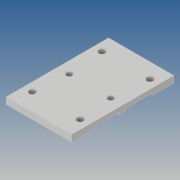
# Autodesk Inventor part: attache_exterieur
Saved by Autodesk Inventor 2019 (Build 230136000, 136)
## iProperties
Created: 2020-07-07
Part Number: attache_exterieur
Material: Générique
Document SubType Name: Modeling
Designer: Theo
Density: 1 g/cm^3
Appearance: Par défaut
Author: Theo
Autodesk Inventor part; units mm, degrees
ref_plane "YZ Plane" through (0, 0, 0) normal (1, 0, 0) x (0, 1, 0)
ref_plane "XZ Plane" through (0, 0, 0) normal (0, 1, 0) x (-1, 0, 0)
ref_plane "XY Plane" through (0, 0, 0) normal (0, 0, 1) x (1, 0, 0)
sketch "Esquisse1" plane through (0, 0, 0) normal (0, 1, 0) x (-1, 0, 0)
  line L0 (0, 0) -> (-60, 0)
  line L1 (-60, 0) -> (-60, 94)
  line L2 (-60, 94) -> (0, 94)
  line L3 (0, 94) -> (0, 0)
  dimension "d0" = 60
  dimension "d1" = 94
  constraints: 8 end point, 2 parallel, 1 horizontal, 1 perpendicular
  measures "d0" distance of L0.start L0.end
  measures "d1" distance of L2.end L0.start
extrude "Extrusion1" add sketch "Esquisse1" along normal blind 6
sketch "Esquisse2" plane through (0, 6, 0) normal (0, 1, 0) x (1, 0, 0)
  line L0 (0, -94) -> (60, -94) projected
  line L1 (60, 0) -> (0, 0) projected
  line L2 (0, 0) -> (0, -94) projected
  line L3 (60, -94) -> (60, 0) projected
  point P0 (8, -78)
  point P1 (52, -78)
  point P2 (52, -14)
  point P3 (8, -14)
  dimension "d4" = 16
  dimension "d5" = 14
  dimension "d6" = 8
  dimension "d7" = 8
  constraints: 2 horizontal alignment, 2 vertical alignment
  measures "d4" distance from line of L0 point (8, -78)
  measures "d5" distance from line of L1 point (8, -14)
  measures "d6" distance from line of L2 point (8, -78)
  measures "d7" distance from line of L3 point (52, -78)
hole "Perçage1" at (8, 6, 78) at (52, 6, 78) at (52, 6, 14) at (8, 6, 14) direction (0, -1, 0) diameter 5.5 end through all clearance for "Vis d'assemblage à tête hexagonale ISO 24017" size "M5" standard "ISO"
sketch "Esquisse4" plane through (0, 0, 0) normal (0, -1, 0) x (1, 0, 0)
  line L0 (0, 94) -> (0, 0) projected
  line L1 (60, 0) -> (60, 94) projected
  point P0 (11, 47)
  point P1 (49, 47)
  point P2 (0, 47)
  dimension "d15" = 11
  dimension "d16" = 11
  constraints: 2 horizontal alignment, 1 midpoint
  measures "d15" distance from line of L0 point (11, 47)
  measures "d16" distance from line of L1 point (49, 47)
hole "Perçage2" at (11, 0, 47) at (49, 0, 47) direction (0, 1, 0) diameter 5 end through all countersink diameter 10 countersink angle 90
sketch "Esquisse5" plane through (0, 0, 0) normal (0, -1, 0) x (1, 0, 0)
  circle A0 centre (11, 47) radius 5 projected
  circle A1 centre (49, 47) radius 5 projected
  circle A2 centre (52, 14) radius 2.75 projected
  circle A3 centre (8, 78) radius 2.75 projected
  circle A4 centre (52, 78) radius 2.75 projected
  circle A5 centre (8, 14) radius 2.75 projected
  line L0 (0, 0) -> (60, 0) projected
  line L1 (60, 0) -> (60, 94) projected
  line L2 (60, 94) -> (0, 94) projected
  line L3 (0, 94) -> (0, 0) projected
  line L4 (60, 0) -> (60, 94) projected
  line L5 (60, 72) -> (0, 72)
  line L6 (0, 72) -> (0, 55)
  line L7 (0, 55) -> (60, 55)
  line L8 (60, 55) -> (60, 72)
  line L9 (60, 39) -> (0, 39)
  line L10 (0, 39) -> (0, 20)
  line L11 (0, 20) -> (60, 20)
  line L12 (60, 20) -> (60, 39)
  dimension "d24" = 6
  dimension "d25" = 6
  dimension "d26" = 8
  dimension "d27" = 8
  constraints: 16 end point, 4 parallel, 4 point on line, 2 horizontal, 2 perpendicular
  measures "d24" distance from line of L5 A4.centre
  measures "d25" distance from line of A2.centre L11
  measures "d26" distance from line of L9 A1.centre
  measures "d27" distance from line of L7 A1.centre
extrude "Extrusion2" cut sketch "Esquisse5" against normal blind 2 contours L3 L9 L1 L11 | L3 L5 L1 L7
chamfer "Chanfrein1" distance 5 angle 45 4 edges at (0, 1, 39) (0, 1, 55) (60, 1, 39) (60, 1, 55)
equation "\"d16\" = d15"
equation "\"d25\" = d24"
equation "\"d27\" = d26"
